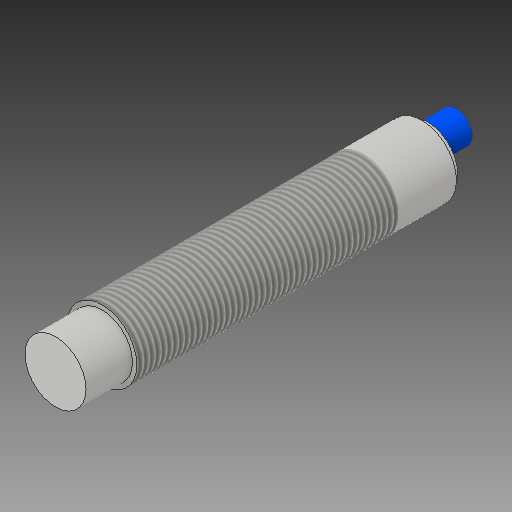
# Autodesk Inventor part: LJ12A3-4-Z-BX
Saved by Autodesk Inventor 2019 (Build 230136000, 136)
## iProperties
Part Number: LJ12A3-4-Z-BX
Material: Типовые
Document SubType Name: Modeling
Designer: SLX
Density: 1 g/cm^3
Appearance: По умолчанию
Mass: 7.02563 g
Surface Area: 27.6639 cm^2
Volume: 7.02563 cm^3
Author: SLX
Autodesk Inventor part; units mm, degrees
ref_plane "YZ Plane" through (0, 0, 0) normal (1, 0, 0) x (0, 1, 0)
ref_plane "XZ Plane" through (0, 0, 0) normal (0, 1, 0) x (-1, 0, 0)
ref_plane "XY Plane" through (0, 0, 0) normal (0, 0, 1) x (1, 0, 0)
sketch "Эскиз1" plane through (0, 0, 0) normal (0, 0, 1) x (1, 0, 0)
  circle A0 centre (0, 0) radius 6
  dimension "d0" = 12
  constraints: 1 centre point, 1 coincident
  measures "d0" diameter of A0
extrude "Выдавливание1" add sketch "Эскиз1" along normal blind 55
sketch "Эскиз2" plane through (0, 0, 55) normal (0, 0, 1) x (1, 0, 0)
  circle A0 centre (0, 0) radius 5.25
  dimension "d3" = 10.5
  constraints: 1 centre point, 1 coincident
  measures "d3" diameter of A0
extrude "Выдавливание2" add sketch "Эскиз2" along normal blind 8
sketch "Эскиз3" plane through (0, 0, 0) normal (0, 0, -1) x (-1, 0, 0)
  circle A0 centre (0, 0) radius 5.25
  dimension "d6" = 10.5
  constraints: 1 centre point, 1 coincident
  measures "d6" diameter of A0
extrude "Выдавливание3" add sketch "Эскиз3" along normal blind 1
thread "Резьба1" size "M12x1" class "6g" standard "ANSI Metric M Profile" length 45
sketch "Эскиз4" plane through (0, 0, -1) normal (0, 0, -1) x (-1, 0, 0)
  circle A0 centre (0, 2) radius 2.75
  circle A1 centre (0, 2) radius 2.5
  point P0 (0, 0)
  dimension "d11" = 5.5
  dimension "d12" = 2
  dimension "d13" = 5
  constraints: 2 centre point, 1 coincident, 1 vertical alignment
  measures "d11" diameter of A0
  measures "d12" distance of point (0, 0) A0.centre
  measures "d13" diameter of A1
extrude "Выдавливание4" add sketch "Эскиз4" along normal blind 5
sketch "Эскиз5" plane through (0, 0, -1) normal (0, 0, -1) x (-1, 0, 0)
  circle A0 centre (0, -3) radius 1.5
  point P0 (0, 0)
  dimension "d16" = 3
  dimension "d17" = 3
  constraints: 1 centre point, 1 vertical alignment
  measures "d16" diameter of A0
  measures "d17" distance of A0.centre point (0, 0)
extrude "Выдавливание5" add sketch "Эскиз5" along normal blind 1
fillet "Сопряжение1" radius 1 1 edges at (1.5, -3, -2)
